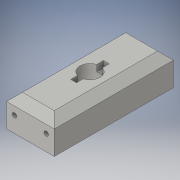
# Autodesk Inventor part: bottom_anchor
Saved by Autodesk Inventor 2016 (Build 200138000, 138)
## iProperties
Created: 2016-02-05
Part Number: bottom_anchor
Material: Generic
Document SubType Name: Modeling
Designer: Matt Ruffner
Density: 1 g/cm^3
Appearance: Default
Author: Matt Ruffner
Autodesk Inventor part; units mm, degrees
ref_plane "YZ Plane" through (0, 0, 0) normal (1, 0, 0) x (0, 1, 0)
ref_plane "XZ Plane" through (0, 0, 0) normal (0, 1, 0) x (-1, 0, 0)
ref_plane "XY Plane" through (0, 0, 0) normal (0, 0, 1) x (1, 0, 0)
sketch "Sketch1" plane through (0, 0, 0) normal (0, 1, 0) x (-1, 0, 0)
  line L0 (8.4018, 18.0616) -> (-10.6482, 18.0616)
  line L1 (-10.6482, 18.0616) -> (-10.6482, -29.5634)
  line L2 (-10.6482, -29.5634) -> (8.4018, -29.5634)
  line L3 (8.4018, -29.5634) -> (8.4018, 18.0616)
  circle A0 centre (-1.1232, -5.7509) radius 4.0005
  point P0 (0, 0)
  dimension "d0" = 19.05
  dimension "d1" = 47.625
  dimension "d2" = 8.001
  constraints: 8 end point, 2 parallel, 1 centre point, 1 horizontal, 1 perpendicular
  measures "d0" distance of L0.start L0.end
  measures "d1" distance of L2.end L0.start
  measures "d2" diameter of A0
extrude "Extrusion1" add sketch "Sketch1" along normal blind 12.7
sketch "Sketch2" plane through (-8.4018, 0, 18.0616) normal (0, 0, 1) x (1, 0, 0)
  line L0 (0, 0) -> (0, 12.7) projected
  line L1 (0, 6.35) -> (18.844, 6.35)
  circle A0 centre (3.175, 6.35) radius 0.889
  circle A1 centre (15.875, 6.35) radius 0.889
  point P0 (8.4018, 0)
  dimension "d5" = 12.7
  dimension "d6" = 3.175
  dimension "d7" = 1.778
  dimension "d8" = 1.778
  constraints: 2 centre point, 2 coincident, 2 end point, 2 point on line, 1 horizontal, 1 midpoint
  measures "d5" distance of point (15.875, 6.35) point (3.175, 6.35)
  measures "d6" distance from line of L0 point (3.175, 6.35)
  measures "d7" diameter of A0
  measures "d8" diameter of A1
extrude "Extrusion2" cut sketch "Sketch2" against normal blind 12.7
sketch "Sketch3" plane through (10.6482, 0, -29.5634) normal (0, 0, -1) x (-1, 0, 0)
  circle A0 centre (3.175, 6.35) radius 0.889 projected
  circle A1 centre (15.875, 6.35) radius 0.889 projected
  point P0 (10.6482, 0)
extrude "Extrusion3" cut sketch "Sketch3" against normal blind 12.7
chamfer "Chamfer1" distance 3.175 angle 45 4 edges at (10.6482, 12.7, -5.7509) (-8.4018, 12.7, -5.7509) (1.1232, 12.7, 18.0616) (1.1232, 12.7, -29.5634)
sketch "Sketch4" plane through (0, 12.7, 0) normal (0, 1, 0) x (1, 0, 0)
  circle A0 centre (1.1232, 5.7509) radius 4.0005 projected
  line L0 (2.2662, 1.7504) -> (2.2662, -0.7896)
  line L1 (2.2662, -0.7896) -> (-0.0198, -0.7896)
  line L2 (-0.0198, -0.7896) -> (-0.0198, 1.7504)
  line L3 (-0.0198, 1.7504) -> (-0.0198, 1.9172)
  line L4 (2.2662, 1.7504) -> (2.2662, 1.9172)
  line L5 (2.2662, 12.2914) -> (2.2662, 9.7514)
  line L6 (-0.0198, 12.2914) -> (2.2662, 12.2914)
  line L7 (-0.0198, 9.7514) -> (-0.0198, 12.2914)
  line L8 (2.2662, 9.7514) -> (2.2662, 9.5847)
  line L9 (-6.1158, 16.8634) -> (-4.3378, 16.8634) projected
  line L10 (-0.0198, 9.7514) -> (-0.0198, 9.5847)
  point P0 (0, 0)
  point P1 (1.1232, 1.7504)
  dimension "d18" = 2.54
  dimension "d21" = 360
  constraints: 20 end point, 5 point on circle, 3 perpendicular, 2 parallel, 2 vertical, 15 other
  measures "d18" distance of L0.start L0.end
extrude "Extrusion4" cut sketch "Sketch4" against normal blind 2.54 contours A0 L10 L7 L6 L5 L8 | L4 L0 L1 L2 L3 A0
body "Solid1"
